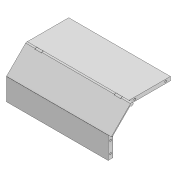
# Autodesk Inventor part: Electronics Housing Main
Saved by Autodesk Inventor 2020 (Build 240168000, 168)
## iProperties
Created: 2021-08-28
Part Number: Electronics Housing Main
Material: Generic
Document SubType Name: Modeling
Designer: Coy
Density: 1 g/cm^3
Appearance: Default
Author: Coy
Autodesk Inventor part; units mm, degrees
ref_plane "YZ Plane" through (0, 0, 0) normal (1, 0, 0) x (0, 1, 0)
ref_plane "XZ Plane" through (0, 0, 0) normal (0, 1, 0) x (-1, 0, 0)
ref_plane "XY Plane" through (0, 0, 0) normal (0, 0, 1) x (1, 0, 0)
sketch "Sketch1" plane through (0, 0, 0) normal (1, 0, 0) x (0, 1, 0)
  line L0 (1, 1) -> (56, 1) construction
  line L1 (56, 1) -> (56, 121) construction
  line L2 (56, 121) -> (1, 121) construction
  line L3 (1, 121) -> (1, 1) construction
  line L4 (80.7487, 174.033) -> (45.3934, 138.6777) construction
  line L5 (45.3934, 138.6777) -> (73.6777, 110.3934) construction
  line L6 (73.6777, 110.3934) -> (109.033, 145.7487) construction
  line L7 (109.033, 145.7487) -> (80.7487, 174.033) construction
  line L8 (59.5355, 124.5355) -> (56, 121) construction
  line L9 (0, 0) -> (125, 0) construction
  line L10 (125, 0) -> (125, 190) construction
  line L11 (125, 190) -> (0, 190) construction
  line L12 (0, 190) -> (0, 0) construction
  line L13 (109.033, 145.7487) -> (80.7487, 174.033) construction
  line L14 (80.7487, 174.033) -> (94.8909, 188.1751) construction
  line L15 (94.8909, 188.1751) -> (123.1751, 159.8909) construction
  line L16 (123.1751, 159.8909) -> (109.033, 145.7487) construction
  line L17 (125, 129.7817) -> (64.7817, 190)
  line L18 (125, 129.7817) -> (125, 0)
  line L19 (125, 0) -> (0, 0)
  line L20 (0, 0) -> (0, 190)
  line L21 (0, 190) -> (64.7817, 190)
  line L22 (66.0244, 193) -> (128, 131.0244)
  line L23 (128, 131.0244) -> (128, -3)
  line L24 (128, -3) -> (-3, -3)
  line L25 (-3, -3) -> (-3, 193)
  line L26 (-3, 193) -> (66.0244, 193)
  line L27 (128, 131.0244) -> (123.1522, 129.0164) construction
  circle A0 centre (123.1522, 129.0164) radius 2.5
  circle A1 centre (123.1522, 129.0164) radius 7.098
  point P0 (122.914, 136.1104)
  point P1 (128, 123.8317)
  dimension "d0" = 55
  dimension "d1" = 120
  dimension "d2" = 50
  dimension "d3" = 40
  dimension "d4" = 135
  dimension "d5" = 135
  dimension "d6" = 5
  dimension "d7" = 125
  dimension "d8" = 190
  dimension "d9" = 1
  dimension "d10" = 1
  dimension "d11" = 20
  dimension "d12" = 3
  dimension "d36" = 5
  dimension "d37" = 14.196
  constraints: 56 end point, 11 perpendicular, 8 parallel, 4 point on line, 2 centre point, 2 coincident, 2 horizontal, 1 collinear, 1 midpoint, 4 other
  measures "d0" distance of L2.end L1.end
  measures "d1" distance of L1.end L0.end
  measures "d2" distance of L4.start L4.end
  measures "d3" distance of L5.end L4.end
  measures "d4" angle of L1 L6
  measures "d5" angle of L1 L8
  measures "d6" distance of L8.start L1.end
  measures "d7" distance of L9.start L9.end
  measures "d8" distance of L11.end L9.start
  measures "d9" distance between parallel lines of L9 L0
  measures "d10" distance between parallel lines of L12 L3
  measures "d11" distance of L4.start L14.end
  measures "d12" distance between parallel lines of L17 L22
  measures "d36" diameter of A0
  measures "d37" diameter of A1
extrude "Extrusion1" add sketch "Sketch1" along normal blind 10
sketch "Sketch2" plane through (10, 0, 0) normal (1, 0, 0) x (0, 0, -1)
  line L0 (-193, -3) -> (3, -3) projected
  line L1 (3, -3) -> (3, 128) projected
  line L2 (3, 128) -> (-123.8317, 128) projected
  line L3 (-136.1104, 122.914) -> (-193, 66.0244) projected
  line L4 (-193, 66.0244) -> (-193, -3) projected
  line L5 (0, 125) -> (0, 0)
  line L6 (0, 0) -> (-190, 0)
  line L7 (-190, 0) -> (-190, 64.7817)
  line L8 (-193, 66.0244) -> (-193, -3) projected
  line L9 (-189.75, 64.6782) -> (-193, 66.0244)
  line L10 (-189.7704, 65.0114) -> (-192.7704, 66.254)
  line L11 (-131.0244, 128) -> (-129.0164, 123.1522) construction
  circle A0 centre (-129.0164, 123.1522) radius 2.5 construction
  circle A1 centre (-129.0164, 123.1522) radius 2.75 construction
  arc A2 (-133.4921, 121.2897) -> (-129.0164, 128) centre (-129.0164, 123.1522) ccw
  line L12 (-131.0244, 128) -> (-193, 66.0244) construction
  line L13 (-133.5692, 120.859) -> (-189.75, 64.6782)
  arc A3 (-133.5692, 120.859) -> (-127.4396, 128) centre (-129.0164, 123.1522) ccw
  line L14 (-129.7817, 125) -> (-126.9796, 125) construction
  line L15 (-124.2653, 125) -> (0, 125)
  line L16 (-190, 64.7817) -> (-133.4921, 121.2897)
  line L17 (-131.7631, 123.0186) -> (-129.7817, 125) construction
  arc A4 (-123.8317, 128) -> (-136.1104, 122.914) centre (-129.0164, 123.1522) ccw projected
  line L18 (-136.1104, 122.914) -> (-131.0244, 128)
  line L19 (3, 128) -> (-123.8317, 128) projected
  line L20 (-131.0244, 128) -> (-123.8317, 128)
  circle A5 centre (-129.0164, 123.1522) radius 4.8478
  circle A6 centre (-129.0164, 123.1522) radius 5.0978
  line L21 (0, 118.0545) -> (-129.0164, 118.0545)
  point P0 (0, 0)
  point P1 (-132.4443, 126.5801)
  dimension "d16" = 0.3
  dimension "d18" = 5
  dimension "d19" = 0.25
  constraints: 28 end point, 7 point on circle, 7 point on line, 5 centre point, 3 coincident, 2 horizontal, 2 parallel, 1 tangent, 1 vertical alignment, 5 other
  measures "d16" distance between parallel lines of L9 L10
  measures "d18" diameter of A0
  measures "d19" radial gap between concentric circles of A0 A1
extrude "Extrusion2" cut sketch "Sketch2" against normal through all contours L3 L10 L16 L9 | L16 A6 L13 L9 | L20 A6 L18 A4 | A3 A6 L16 A2 L20 | L20 A6 | A6 L18 | A5 L18 A6 L20 | A6 L18 L20
sketch "Sketch3" plane through (10, 0, 0) normal (1, 0, 0) x (0, 0, -1)
  line L0 (-193, -3) -> (3, -3)
  line L1 (3, -3) -> (3, 128)
  line L2 (3, 128) -> (-131.0244, 128)
  line L3 (-131.0244, 128) -> (-192.7704, 66.254)
  line L4 (-193, 66.0244) -> (-193, -3)
  line L5 (0, 125) -> (0, 0)
  line L6 (0, 0) -> (-190, 0)
  line L7 (-190, 0) -> (-190, 64.7817)
  line L8 (-193, 66.0244) -> (-193, -3)
  line L9 (-189.75, 64.6782) -> (-193, 66.0244)
  line L10 (-189.7704, 65.0114) -> (-192.7704, 66.254)
  line L11 (-131.0244, 128) -> (-129.0164, 123.1522) construction
  circle A0 centre (-129.0164, 123.1522) radius 2.5 construction
  circle A1 centre (-129.0164, 123.1522) radius 2.75 construction
  arc A2 (-133.4921, 121.2897) -> (-129.0164, 128) centre (-129.0164, 123.1522) ccw
  line L12 (-131.0244, 128) -> (-193, 66.0244) construction
  line L13 (-133.5692, 120.859) -> (-189.75, 64.6782)
  arc A3 (-133.5692, 120.859) -> (-127.4396, 128) centre (-129.0164, 123.1522) ccw
  line L14 (-129.7817, 125) -> (-126.9796, 125) construction
  line L15 (-122.1634, 125) -> (0, 125)
  line L16 (-189.7704, 65.0114) -> (-133.4921, 121.2897)
  line L17 (-131.7631, 123.0186) -> (-129.7817, 125) construction
  arc A4 (-135.0362, 119.392) -> (-122.1634, 125) centre (-129.0164, 123.1522) ccw
  arc A5 (-133.4921, 121.2897) -> (-132.4443, 126.5801) centre (-129.0164, 123.1522) ccw projected
  line L18 (0, 116.0545) -> (-129.0164, 116.0545)
  point P0 (0, 0)
  point P1 (0, 0)
  dimension "d25" = 0.3
  dimension "d26" = 5
  dimension "d27" = 0.25
  dimension "d28" = 2
  constraints: 38 end point, 9 point on circle, 6 point on line, 5 centre point, 2 tangent, 1 coincident, 1 horizontal, 1 parallel, 2 other
  measures "d25" distance between parallel lines of L9 L10
  measures "d26" diameter of A0
  measures "d27" radial gap between concentric circles of A0 A1
  measures "d28" radial gap between concentric circles of A3 A4
extrude "Extrusion3" add sketch "Sketch3" along normal blind 20 contours L4 L9 L7 L6 L5 L15 A4 L13 A3 L2 L1 L0 | L18 A4 L15 L5 | A2 L16 L10 L3 A5
sketch "Sketch4" plane through (30, 0, 0) normal (1, 0, 0) x (0, 0, -1)
  line L0 (-193, -3) -> (3, -3)
  line L1 (3, -3) -> (3, 128)
  line L2 (3, 128) -> (-123.8317, 128)
  line L3 (-136.1104, 122.914) -> (-193, 66.0244)
  line L4 (-193, 66.0244) -> (-193, -3)
  line L5 (0, 125) -> (0, 0)
  line L6 (0, 0) -> (-190, 0)
  line L7 (-190, 0) -> (-190, 64.7817)
  line L8 (-193, 66.0244) -> (-193, -3)
  line L9 (-189.75, 64.6782) -> (-193, 66.0244)
  line L10 (-189.7704, 65.0114) -> (-192.7704, 66.254)
  line L11 (-131.0244, 128) -> (-129.0164, 123.1522) construction
  circle A0 centre (-129.0164, 123.1522) radius 2.5
  circle A1 centre (-129.0164, 123.1522) radius 2.75 construction
  arc A2 (-133.4921, 121.2897) -> (-129.0164, 128) centre (-129.0164, 123.1522) ccw
  line L12 (-131.0244, 128) -> (-193, 66.0244) construction
  line L13 (-133.5692, 120.859) -> (-189.75, 64.6782)
  arc A3 (-133.5692, 120.859) -> (-127.4396, 128) centre (-129.0164, 123.1522) ccw
  line L14 (-129.7817, 125) -> (-126.9796, 125) construction
  line L15 (-124.2653, 125) -> (0, 125)
  line L16 (-190, 64.7817) -> (-133.4921, 121.2897)
  line L17 (-131.7631, 123.0186) -> (-129.7817, 125) construction
  arc A4 (-123.8317, 128) -> (-136.1104, 122.914) centre (-129.0164, 123.1522) ccw
  line L18 (-136.1104, 122.914) -> (-131.0244, 128)
  line L19 (3, 128) -> (-123.8317, 128)
  line L20 (-131.0244, 128) -> (-123.8317, 128)
  circle A5 centre (-129.0164, 123.1522) radius 4.8478
  circle A6 centre (-129.0164, 123.1522) radius 5.0978
  line L21 (0, 116.0545) -> (0, 0) projected
  line L22 (0, 0) -> (-190, 0) projected
  line L23 (-190, 0) -> (-190, 64.7817) projected
  line L24 (-190, 64.7817) -> (-193, 66.0244) projected
  line L25 (-193, 66.0244) -> (-193, -3) projected
  line L26 (-193, -3) -> (3, -3) projected
  line L27 (3, -3) -> (3, 128) projected
  line L28 (3, 128) -> (-127.4396, 128) projected
  arc A7 (-133.5692, 120.859) -> (-127.4396, 128) centre (-129.0164, 123.1522) ccw projected
  line L29 (-133.5692, 120.859) -> (-135.0362, 119.392) projected
  arc A8 (-135.0362, 119.392) -> (-129.0164, 116.0545) centre (-129.0164, 123.1522) ccw projected
  arc A9 (-133.4921, 121.2897) -> (-132.4443, 126.5801) centre (-129.0164, 123.1522) ccw projected
  line L30 (-132.4443, 126.5801) -> (-192.7704, 66.254) projected
  line L31 (-192.7704, 66.254) -> (-189.7704, 65.0114) projected
  line L32 (-189.7704, 65.0114) -> (-133.4921, 121.2897) projected
  line L33 (-129.0164, 116.0545) -> (0, 116.0545) projected
  point P0 (0, 0)
  point P1 (-127.4396, 128)
  point P2 (-122.1634, 125)
  point P3 (-133.6825, 121.0993)
  point P4 (-133.5592, 125.4651)
  point P5 (0, 116.0545)
  point P6 (0, 66.508)
  dimension "d38" = 0.3
  dimension "d39" = 5
  dimension "d40" = 0.25
  constraints: 42 end point, 9 point on circle, 7 centre point, 6 point on line, 3 coincident, 1 concentric, 1 horizontal, 1 parallel, 1 tangent, 2 other
  measures "d38" distance between parallel lines of L9 L10
  measures "d39" diameter of A0
  measures "d40" radial gap between concentric circles of A0 A1
extrude "Extrusion4" add sketch "Sketch4" along normal blind 0.35 contours L4 L9 L7 L6 L5 L15 A3 L20 L2 L1 L0 | L3 L18 A6 L16 L10 | L13 A3 L15 L5 L33 A8 | A0
sketch "Sketch5" plane through (30.35, 0, 0) normal (1, 0, 0) x (0, 0, -1)
  line L0 (-193, -3) -> (3, -3)
  line L1 (3, -3) -> (3, 128)
  line L2 (3, 128) -> (-123.8317, 128)
  line L3 (-136.1104, 122.914) -> (-193, 66.0244)
  line L4 (-193, 66.0244) -> (-193, -3)
  line L5 (0, 125) -> (0, 0)
  line L6 (0, 0) -> (-190, 0)
  line L7 (-190, 0) -> (-190, 64.7817)
  line L8 (-193, 66.0244) -> (-193, -3)
  line L9 (-189.75, 64.6782) -> (-193, 66.0244)
  line L10 (-189.7704, 65.0114) -> (-192.7704, 66.254)
  line L11 (-131.0244, 128) -> (-129.0164, 123.1522) construction
  circle A0 centre (-129.0164, 123.1522) radius 2.5
  circle A1 centre (-129.0164, 123.1522) radius 2.75
  arc A2 (-133.4921, 121.2897) -> (-129.0164, 128) centre (-129.0164, 123.1522) ccw
  line L12 (-131.0244, 128) -> (-193, 66.0244) construction
  line L13 (-133.5692, 120.859) -> (-189.75, 64.6782)
  arc A3 (-133.5692, 120.859) -> (-127.4396, 128) centre (-129.0164, 123.1522) ccw
  line L14 (-129.7817, 125) -> (-126.9796, 125) construction
  line L15 (-124.2653, 125) -> (0, 125)
  line L16 (-190, 64.7817) -> (-133.4921, 121.2897)
  line L17 (-131.7631, 123.0186) -> (-129.7817, 125) construction
  arc A4 (-123.8317, 128) -> (-136.1104, 122.914) centre (-129.0164, 123.1522) ccw
  line L18 (-136.1104, 122.914) -> (-131.0244, 128)
  line L19 (3, 128) -> (-123.8317, 128)
  line L20 (-131.0244, 128) -> (-123.8317, 128)
  circle A5 centre (-129.0164, 123.1522) radius 4.8478
  circle A6 centre (-129.0164, 123.1522) radius 5.0978
  line L21 (0, 125) -> (0, 0)
  line L22 (0, 0) -> (-190, 0)
  line L23 (-190, 0) -> (-190, 64.7817)
  line L24 (-190, 64.7817) -> (-193, 66.0244)
  line L25 (-193, 66.0244) -> (-193, -3)
  line L26 (-193, -3) -> (3, -3)
  line L27 (3, -3) -> (3, 128)
  line L28 (3, 128) -> (-127.4396, 128)
  arc A7 (-133.5692, 120.859) -> (-127.4396, 128) centre (-129.0164, 123.1522) ccw
  line L29 (-133.3825, 121.0457) -> (-135.0362, 119.392)
  arc A8 (-135.0362, 119.392) -> (-122.1634, 125) centre (-129.0164, 123.1522) ccw
  line L30 (-122.1634, 125) -> (0, 125)
  arc A9 (-133.4921, 121.2897) -> (-132.4443, 126.5801) centre (-129.0164, 123.1522) ccw
  line L31 (-132.4443, 126.5801) -> (-192.7704, 66.254)
  line L32 (-192.7704, 66.254) -> (-189.7704, 65.0114)
  line L33 (-189.7704, 65.0114) -> (-133.4921, 121.2897)
  line L34 (-127.4396, 128) -> (-127.5334, 127.7676)
  line L35 (-129.0164, 116.0545) -> (0, 116.0545) projected
  point P0 (0, 0)
  point P1 (0, 0)
  point P2 (-127.4396, 128)
  point P3 (-122.1634, 125)
  point P4 (-133.6825, 121.0993)
  point P5 (-133.5592, 125.4651)
  point P6 (-127.4396, 128)
  point P7 (-122.1634, 125)
  point P8 (-133.6825, 121.0993)
  point P9 (-133.5592, 125.4651)
  dimension "d43" = 0.3
  dimension "d44" = 5
  dimension "d45" = 0.25
  dimension "d46" = 112
  constraints: 70 end point, 16 point on circle, 9 centre point, 7 point on line, 3 coincident, 1 concentric, 1 horizontal, 1 parallel, 1 tangent, 5 other
  measures "d43" distance between parallel lines of L9 L10
  measures "d44" diameter of A0
  measures "d45" radial gap between concentric circles of A0 A1
  measures "d46" angle of L20 L34
extrude "Extrusion5" add sketch "Sketch5" along normal blind 20 contours L4 L9 L7 L6 L5 L15 A3 L20 L2 L1 L0 | L3 L18 A6 L16 L10 | A3 L29 A2 L34 | L13 A3 L15 A8 | A2 A5 | L35 A8 L15 L5 | A0
sketch "Sketch6" plane through (50.35, 0, 0) normal (1, 0, 0) x (0, 0, -1)
  line L0 (-193, -3) -> (3, -3)
  line L1 (3, -3) -> (3, 128)
  line L2 (3, 128) -> (-123.8317, 128)
  line L3 (-136.1104, 122.914) -> (-193, 66.0244)
  line L4 (-193, 66.0244) -> (-193, -3)
  line L5 (0, 125) -> (0, 0)
  line L6 (0, 0) -> (-190, 0)
  line L7 (-190, 0) -> (-190, 64.7817)
  line L8 (-193, 66.0244) -> (-193, -3)
  line L9 (-189.75, 64.6782) -> (-193, 66.0244)
  line L10 (-189.7704, 65.0114) -> (-192.7704, 66.254)
  line L11 (-131.0244, 128) -> (-129.0164, 123.1522) construction
  circle A0 centre (-129.0164, 123.1522) radius 2.5
  circle A1 centre (-129.0164, 123.1522) radius 2.75
  arc A2 (-133.4921, 121.2897) -> (-129.0164, 128) centre (-129.0164, 123.1522) ccw
  line L12 (-131.0244, 128) -> (-193, 66.0244) construction
  line L13 (-133.5692, 120.859) -> (-189.75, 64.6782)
  arc A3 (-133.5692, 120.859) -> (-127.4396, 128) centre (-129.0164, 123.1522) ccw
  line L14 (-129.7817, 125) -> (-126.9796, 125) construction
  line L15 (-124.2653, 125) -> (0, 125)
  line L16 (-190, 64.7817) -> (-133.4921, 121.2897)
  line L17 (-131.7631, 123.0186) -> (-129.7817, 125) construction
  arc A4 (-123.8317, 128) -> (-136.1104, 122.914) centre (-129.0164, 123.1522) ccw
  line L18 (-136.1104, 122.914) -> (-131.0244, 128)
  line L19 (3, 128) -> (-123.8317, 128)
  line L20 (-131.0244, 128) -> (-123.8317, 128)
  circle A5 centre (-129.0164, 123.1522) radius 4.8478
  circle A6 centre (-129.0164, 123.1522) radius 5.0978
  line L21 (0, 125) -> (0, 0)
  line L22 (0, 0) -> (-190, 0)
  line L23 (-190, 0) -> (-190, 64.7817)
  line L24 (-190, 64.7817) -> (-193, 66.0244)
  line L25 (-193, 66.0244) -> (-193, -3)
  line L26 (-193, -3) -> (3, -3)
  line L27 (3, -3) -> (3, 128)
  line L28 (3, 128) -> (-127.4396, 128)
  arc A7 (-133.5692, 120.859) -> (-127.4396, 128) centre (-129.0164, 123.1522) ccw
  line L29 (-133.3825, 121.0457) -> (-135.0362, 119.392)
  arc A8 (-135.0362, 119.392) -> (-122.1634, 125) centre (-129.0164, 123.1522) ccw
  line L30 (-122.1634, 125) -> (0, 125)
  arc A9 (-133.4921, 121.2897) -> (-132.4443, 126.5801) centre (-129.0164, 123.1522) ccw
  line L31 (-132.4443, 126.5801) -> (-192.7704, 66.254)
  line L32 (-192.7704, 66.254) -> (-189.7704, 65.0114)
  line L33 (-189.7704, 65.0114) -> (-133.4921, 121.2897)
  line L34 (-127.4396, 128) -> (-127.5334, 127.7676)
  line L35 (-129.0164, 116.0545) -> (0, 116.0545) projected
  point P0 (0, 0)
  point P1 (0, 0)
  point P2 (0, 0)
  point P3 (-127.4396, 128)
  point P4 (-122.1634, 125)
  point P5 (-133.6825, 121.0993)
  point P6 (-133.5592, 125.4651)
  point P7 (-127.4396, 128)
  point P8 (-122.1634, 125)
  point P9 (-133.6825, 121.0993)
  point P10 (-133.5592, 125.4651)
  point P11 (-127.4396, 128)
  point P12 (-122.1634, 125)
  point P13 (-133.6825, 121.0993)
  point P14 (-133.5592, 125.4651)
  dimension "d49" = 0.3
  dimension "d50" = 5
  dimension "d51" = 0.25
  dimension "d52" = 112
  constraints: 70 end point, 16 point on circle, 9 centre point, 7 point on line, 3 coincident, 1 concentric, 1 horizontal, 1 parallel, 1 tangent, 5 other
  measures "d49" distance between parallel lines of L9 L10
  measures "d50" diameter of A0
  measures "d51" radial gap between concentric circles of A0 A1
  measures "d52" angle of L20 L34
extrude "Extrusion6" add sketch "Sketch6" along normal blind 0.35 contours L4 L9 L7 L6 L5 L15 A3 L20 L2 L1 L0 | L3 L18 A6 L16 L10 | L13 A3 L15 A8 | L35 A8 L15 L5 | A0
sketch "Sketch7" plane through (50.7, 0, 0) normal (1, 0, 0) x (0, 0, -1)
  line L0 (-193, -3) -> (3, -3)
  line L1 (3, -3) -> (3, 128)
  line L2 (3, 128) -> (-123.8317, 128)
  line L3 (-136.1104, 122.914) -> (-193, 66.0244)
  line L4 (-193, 66.0244) -> (-193, -3)
  line L5 (0, 125) -> (0, 0)
  line L6 (0, 0) -> (-190, 0)
  line L7 (-190, 0) -> (-190, 64.7817)
  line L8 (-193, 66.0244) -> (-193, -3)
  line L9 (-189.75, 64.6782) -> (-193, 66.0244)
  line L10 (-189.7704, 65.0114) -> (-192.7704, 66.254)
  line L11 (-131.0244, 128) -> (-129.0164, 123.1522) construction
  circle A0 centre (-129.0164, 123.1522) radius 2.5
  circle A1 centre (-129.0164, 123.1522) radius 2.75
  arc A2 (-133.4921, 121.2897) -> (-129.0164, 128) centre (-129.0164, 123.1522) ccw
  line L12 (-131.0244, 128) -> (-193, 66.0244) construction
  line L13 (-133.5692, 120.859) -> (-189.75, 64.6782)
  arc A3 (-133.5692, 120.859) -> (-127.4396, 128) centre (-129.0164, 123.1522) ccw
  line L14 (-129.7817, 125) -> (-126.9796, 125) construction
  line L15 (-124.2653, 125) -> (0, 125)
  line L16 (-190, 64.7817) -> (-133.4921, 121.2897)
  line L17 (-131.7631, 123.0186) -> (-129.7817, 125) construction
  arc A4 (-123.8317, 128) -> (-136.1104, 122.914) centre (-129.0164, 123.1522) ccw
  line L18 (-136.1104, 122.914) -> (-131.0244, 128)
  line L19 (3, 128) -> (-123.8317, 128)
  line L20 (-131.0244, 128) -> (-123.8317, 128)
  circle A5 centre (-129.0164, 123.1522) radius 4.8478
  circle A6 centre (-129.0164, 123.1522) radius 5.0978
  line L21 (0, 125) -> (0, 0)
  line L22 (0, 0) -> (-190, 0)
  line L23 (-190, 0) -> (-190, 64.7817)
  line L24 (-190, 64.7817) -> (-193, 66.0244)
  line L25 (-193, 66.0244) -> (-193, -3)
  line L26 (-193, -3) -> (3, -3)
  line L27 (3, -3) -> (3, 128)
  line L28 (3, 128) -> (-127.4396, 128)
  arc A7 (-133.5692, 120.859) -> (-127.4396, 128) centre (-129.0164, 123.1522) ccw
  line L29 (-133.3825, 121.0457) -> (-135.0362, 119.392)
  arc A8 (-135.0362, 119.392) -> (-122.1634, 125) centre (-129.0164, 123.1522) ccw
  line L30 (-122.1634, 125) -> (0, 125)
  arc A9 (-133.4921, 121.2897) -> (-132.4443, 126.5801) centre (-129.0164, 123.1522) ccw
  line L31 (-132.4443, 126.5801) -> (-192.7704, 66.254)
  line L32 (-192.7704, 66.254) -> (-189.7704, 65.0114)
  line L33 (-189.7704, 65.0114) -> (-133.4921, 121.2897)
  line L34 (-127.4396, 128) -> (-127.5334, 127.7676)
  line L35 (-129.0164, 116.0545) -> (0, 116.0545) projected
  point P0 (0, 0)
  point P1 (0, 0)
  point P2 (0, 0)
  point P3 (0, 0)
  point P4 (-127.4396, 128)
  point P5 (-122.1634, 125)
  point P6 (-133.6825, 121.0993)
  point P7 (-133.5592, 125.4651)
  point P8 (-127.4396, 128)
  point P9 (-122.1634, 125)
  point P10 (-133.6825, 121.0993)
  point P11 (-133.5592, 125.4651)
  point P12 (-127.4396, 128)
  point P13 (-122.1634, 125)
  point P14 (-133.6825, 121.0993)
  point P15 (-133.5592, 125.4651)
  point P16 (-127.4396, 128)
  point P17 (-122.1634, 125)
  dimension "d55" = 0.3
  dimension "d56" = 5
  dimension "d57" = 0.25
  dimension "d58" = 112
  constraints: 70 end point, 16 point on circle, 9 centre point, 7 point on line, 3 coincident, 1 concentric, 1 horizontal, 1 parallel, 1 tangent, 5 other
  measures "d55" distance between parallel lines of L9 L10
  measures "d56" diameter of A0
  measures "d57" radial gap between concentric circles of A0 A1
  measures "d58" angle of L20 L34
extrude "Extrusion7" add sketch "Sketch7" along normal blind 228.6 contours L4 L9 L7 L6 L5 L15 A3 L20 L2 L1 L0 | L3 L18 A6 L16 L10 | L18 A5 L16 A6 | L13 A3 L15 A8 | A2 A5 | L35 A8 L15 L5 | A0 | A1
sketch "Sketch8" plane through (279.3, 0, 0) normal (1, 0, 0) x (0, 0, -1)
  line L0 (-193, -3) -> (3, -3)
  line L1 (3, -3) -> (3, 128)
  line L2 (3, 128) -> (-123.8317, 128)
  line L3 (-136.1104, 122.914) -> (-193, 66.0244)
  line L4 (-193, 66.0244) -> (-193, -3)
  line L5 (0, 125) -> (0, 0)
  line L6 (0, 0) -> (-190, 0)
  line L7 (-190, 0) -> (-190, 64.7817)
  line L8 (-193, 66.0244) -> (-193, -3)
  line L9 (-189.75, 64.6782) -> (-193, 66.0244)
  line L10 (-189.7704, 65.0114) -> (-192.7704, 66.254)
  line L11 (-131.0244, 128) -> (-129.0164, 123.1522) construction
  circle A0 centre (-129.0164, 123.1522) radius 2.5
  circle A1 centre (-129.0164, 123.1522) radius 2.75
  arc A2 (-133.4921, 121.2897) -> (-129.0164, 128) centre (-129.0164, 123.1522) ccw
  line L12 (-131.0244, 128) -> (-193, 66.0244) construction
  line L13 (-133.5692, 120.859) -> (-189.75, 64.6782)
  arc A3 (-133.5692, 120.859) -> (-127.4396, 128) centre (-129.0164, 123.1522) ccw
  line L14 (-129.7817, 125) -> (-126.9796, 125) construction
  line L15 (-124.2653, 125) -> (0, 125)
  line L16 (-190, 64.7817) -> (-133.4921, 121.2897)
  line L17 (-131.7631, 123.0186) -> (-129.7817, 125) construction
  arc A4 (-123.8317, 128) -> (-136.1104, 122.914) centre (-129.0164, 123.1522) ccw
  line L18 (-136.1104, 122.914) -> (-131.0244, 128)
  line L19 (3, 128) -> (-123.8317, 128)
  line L20 (-131.0244, 128) -> (-123.8317, 128)
  circle A5 centre (-129.0164, 123.1522) radius 4.8478
  circle A6 centre (-129.0164, 123.1522) radius 5.0978
  line L21 (0, 125) -> (0, 0)
  line L22 (0, 0) -> (-190, 0)
  line L23 (-190, 0) -> (-190, 64.7817)
  line L24 (-190, 64.7817) -> (-193, 66.0244)
  line L25 (-193, 66.0244) -> (-193, -3)
  line L26 (-193, -3) -> (3, -3)
  line L27 (3, -3) -> (3, 128)
  line L28 (3, 128) -> (-127.4396, 128)
  arc A7 (-133.5692, 120.859) -> (-127.4396, 128) centre (-129.0164, 123.1522) ccw
  line L29 (-133.3825, 121.0457) -> (-135.0362, 119.392)
  arc A8 (-135.0362, 119.392) -> (-122.1634, 125) centre (-129.0164, 123.1522) ccw
  line L30 (-122.1634, 125) -> (0, 125)
  arc A9 (-133.4921, 121.2897) -> (-132.4443, 126.5801) centre (-129.0164, 123.1522) ccw
  line L31 (-132.4443, 126.5801) -> (-192.7704, 66.254)
  line L32 (-192.7704, 66.254) -> (-189.7704, 65.0114)
  line L33 (-189.7704, 65.0114) -> (-133.4921, 121.2897)
  line L34 (-127.4396, 128) -> (-127.5334, 127.7676)
  line L35 (-129.0164, 116.0545) -> (0, 116.0545) projected
  point P0 (0, 0)
  point P1 (0, 0)
  point P2 (0, 0)
  point P3 (0, 0)
  point P4 (-127.4396, 128)
  point P5 (-122.1634, 125)
  point P6 (-133.6825, 121.0993)
  point P7 (-133.5592, 125.4651)
  point P8 (-127.4396, 128)
  point P9 (-122.1634, 125)
  point P10 (-133.6825, 121.0993)
  point P11 (-133.5592, 125.4651)
  point P12 (-127.4396, 128)
  point P13 (-122.1634, 125)
  point P14 (-133.6825, 121.0993)
  point P15 (-133.5592, 125.4651)
  point P16 (-133.6825, 121.0993)
  point P17 (-133.5592, 125.4651)
  point P18 (-127.4396, 128)
  point P19 (-122.1634, 125)
  dimension "d61" = 0.3
  dimension "d62" = 5
  dimension "d63" = 0.25
  dimension "d64" = 112
  constraints: 70 end point, 16 point on circle, 9 centre point, 7 point on line, 3 coincident, 1 concentric, 1 horizontal, 1 parallel, 1 tangent, 5 other
  measures "d61" distance between parallel lines of L9 L10
  measures "d62" diameter of A0
  measures "d63" radial gap between concentric circles of A0 A1
  measures "d64" angle of L20 L34
extrude "Extrusion8" add sketch "Sketch8" along normal blind 0.35 contours L4 L9 L7 L6 L5 L15 A3 L20 L2 L1 L0 | L3 L18 A6 L16 L10 | L13 A3 L15 A8 | L35 A8 L15 L5 | A0
sketch "Sketch9" plane through (279.65, 0, 0) normal (1, 0, 0) x (0, 0, -1)
  line L0 (-193, -3) -> (3, -3)
  line L1 (3, -3) -> (3, 128)
  line L2 (3, 128) -> (-123.8317, 128)
  line L3 (-136.1104, 122.914) -> (-193, 66.0244)
  line L4 (-193, 66.0244) -> (-193, -3)
  line L5 (0, 125) -> (0, 0)
  line L6 (0, 0) -> (-190, 0)
  line L7 (-190, 0) -> (-190, 64.7817)
  line L8 (-193, 66.0244) -> (-193, -3)
  line L9 (-189.75, 64.6782) -> (-193, 66.0244)
  line L10 (-189.7704, 65.0114) -> (-192.7704, 66.254)
  line L11 (-131.0244, 128) -> (-129.0164, 123.1522) construction
  circle A0 centre (-129.0164, 123.1522) radius 2.5
  circle A1 centre (-129.0164, 123.1522) radius 2.75
  arc A2 (-133.4921, 121.2897) -> (-129.0164, 128) centre (-129.0164, 123.1522) ccw
  line L12 (-131.0244, 128) -> (-193, 66.0244) construction
  line L13 (-133.5692, 120.859) -> (-189.75, 64.6782)
  arc A3 (-133.5692, 120.859) -> (-127.4396, 128) centre (-129.0164, 123.1522) ccw
  line L14 (-129.7817, 125) -> (-126.9796, 125) construction
  line L15 (-124.2653, 125) -> (0, 125)
  line L16 (-190, 64.7817) -> (-133.4921, 121.2897)
  line L17 (-131.7631, 123.0186) -> (-129.7817, 125) construction
  arc A4 (-123.8317, 128) -> (-136.1104, 122.914) centre (-129.0164, 123.1522) ccw
  line L18 (-136.1104, 122.914) -> (-131.0244, 128)
  line L19 (3, 128) -> (-123.8317, 128)
  line L20 (-131.0244, 128) -> (-123.8317, 128)
  circle A5 centre (-129.0164, 123.1522) radius 4.8478
  circle A6 centre (-129.0164, 123.1522) radius 5.0978
  line L21 (0, 125) -> (0, 0)
  line L22 (0, 0) -> (-190, 0)
  line L23 (-190, 0) -> (-190, 64.7817)
  line L24 (-190, 64.7817) -> (-193, 66.0244)
  line L25 (-193, 66.0244) -> (-193, -3)
  line L26 (-193, -3) -> (3, -3)
  line L27 (3, -3) -> (3, 128)
  line L28 (3, 128) -> (-127.4396, 128)
  arc A7 (-133.5692, 120.859) -> (-127.4396, 128) centre (-129.0164, 123.1522) ccw
  line L29 (-133.3825, 121.0457) -> (-135.0362, 119.392)
  arc A8 (-135.0362, 119.392) -> (-122.1634, 125) centre (-129.0164, 123.1522) ccw
  line L30 (-122.1634, 125) -> (0, 125)
  arc A9 (-133.4921, 121.2897) -> (-132.4443, 126.5801) centre (-129.0164, 123.1522) ccw
  line L31 (-132.4443, 126.5801) -> (-192.7704, 66.254)
  line L32 (-192.7704, 66.254) -> (-189.7704, 65.0114)
  line L33 (-189.7704, 65.0114) -> (-133.4921, 121.2897)
  line L34 (-127.4396, 128) -> (-127.5334, 127.7676)
  line L35 (-129.0164, 116.0545) -> (0, 116.0545) projected
  point P0 (0, 0)
  point P1 (0, 0)
  point P2 (0, 0)
  point P3 (0, 0)
  point P4 (0, 0)
  point P5 (-127.4396, 128)
  point P6 (-122.1634, 125)
  point P7 (-133.6825, 121.0993)
  point P8 (-133.5592, 125.4651)
  point P9 (-127.4396, 128)
  point P10 (-122.1634, 125)
  point P11 (-133.6825, 121.0993)
  point P12 (-133.5592, 125.4651)
  point P13 (-127.4396, 128)
  point P14 (-122.1634, 125)
  point P15 (-133.6825, 121.0993)
  point P16 (-133.5592, 125.4651)
  point P17 (-133.6825, 121.0993)
  point P18 (-133.5592, 125.4651)
  point P19 (-127.4396, 128)
  point P20 (-122.1634, 125)
  point P21 (-133.6825, 121.0993)
  point P22 (-133.5592, 125.4651)
  point P23 (-127.4396, 128)
  point P24 (-122.1634, 125)
  dimension "d67" = 0.3
  dimension "d68" = 5
  dimension "d69" = 0.25
  dimension "d70" = 112
  constraints: 70 end point, 16 point on circle, 9 centre point, 7 point on line, 3 coincident, 1 concentric, 1 horizontal, 1 parallel, 1 tangent, 5 other
  measures "d67" distance between parallel lines of L9 L10
  measures "d68" diameter of A0
  measures "d69" radial gap between concentric circles of A0 A1
  measures "d70" angle of L20 L34
extrude "Extrusion9" add sketch "Sketch9" along normal blind 20 contours L4 L9 L7 L6 L5 L15 A3 L20 L2 L1 L0 | L3 L18 A6 L16 L10 | A3 L29 A2 L34 | L13 A3 L15 A8 | A2 A5 | L35 A8 L15 L5 | A0
sketch "Sketch10" plane through (299.65, 0, 0) normal (1, 0, 0) x (0, 0, -1)
  line L0 (-193, -3) -> (3, -3)
  line L1 (3, -3) -> (3, 128)
  line L2 (3, 128) -> (-123.8317, 128)
  line L3 (-136.1104, 122.914) -> (-193, 66.0244)
  line L4 (-193, 66.0244) -> (-193, -3)
  line L5 (0, 125) -> (0, 0)
  line L6 (0, 0) -> (-190, 0)
  line L7 (-190, 0) -> (-190, 64.7817)
  line L8 (-193, 66.0244) -> (-193, -3)
  line L9 (-189.75, 64.6782) -> (-193, 66.0244)
  line L10 (-189.7704, 65.0114) -> (-192.7704, 66.254)
  line L11 (-131.0244, 128) -> (-129.0164, 123.1522) construction
  circle A0 centre (-129.0164, 123.1522) radius 2.5
  circle A1 centre (-129.0164, 123.1522) radius 2.75
  arc A2 (-133.4921, 121.2897) -> (-129.0164, 128) centre (-129.0164, 123.1522) ccw
  line L12 (-131.0244, 128) -> (-193, 66.0244) construction
  line L13 (-133.5692, 120.859) -> (-189.75, 64.6782)
  arc A3 (-133.5692, 120.859) -> (-127.4396, 128) centre (-129.0164, 123.1522) ccw
  line L14 (-129.7817, 125) -> (-126.9796, 125) construction
  line L15 (-124.2653, 125) -> (0, 125)
  line L16 (-190, 64.7817) -> (-133.4921, 121.2897)
  line L17 (-131.7631, 123.0186) -> (-129.7817, 125) construction
  arc A4 (-123.8317, 128) -> (-136.1104, 122.914) centre (-129.0164, 123.1522) ccw
  line L18 (-136.1104, 122.914) -> (-131.0244, 128)
  line L19 (3, 128) -> (-123.8317, 128)
  line L20 (-131.0244, 128) -> (-123.8317, 128)
  circle A5 centre (-129.0164, 123.1522) radius 4.8478
  circle A6 centre (-129.0164, 123.1522) radius 5.0978
  line L21 (0, 125) -> (0, 0)
  line L22 (0, 0) -> (-190, 0)
  line L23 (-190, 0) -> (-190, 64.7817)
  line L24 (-190, 64.7817) -> (-193, 66.0244)
  line L25 (-193, 66.0244) -> (-193, -3)
  line L26 (-193, -3) -> (3, -3)
  line L27 (3, -3) -> (3, 128)
  line L28 (3, 128) -> (-127.4396, 128)
  arc A7 (-133.5692, 120.859) -> (-127.4396, 128) centre (-129.0164, 123.1522) ccw
  line L29 (-133.3825, 121.0457) -> (-135.0362, 119.392)
  arc A8 (-135.0362, 119.392) -> (-122.1634, 125) centre (-129.0164, 123.1522) ccw
  line L30 (-122.1634, 125) -> (0, 125)
  arc A9 (-133.4921, 121.2897) -> (-132.4443, 126.5801) centre (-129.0164, 123.1522) ccw
  line L31 (-132.4443, 126.5801) -> (-192.7704, 66.254)
  line L32 (-192.7704, 66.254) -> (-189.7704, 65.0114)
  line L33 (-189.7704, 65.0114) -> (-133.4921, 121.2897)
  line L34 (-127.4396, 128) -> (-127.5334, 127.7676)
  line L35 (-129.0164, 116.0545) -> (0, 116.0545) projected
  point P0 (0, 0)
  point P1 (0, 0)
  point P2 (0, 0)
  point P3 (0, 0)
  point P4 (0, 0)
  point P5 (-127.4396, 128)
  point P6 (-122.1634, 125)
  point P7 (-133.6825, 121.0993)
  point P8 (-133.5592, 125.4651)
  point P9 (-127.4396, 128)
  point P10 (-122.1634, 125)
  point P11 (-133.6825, 121.0993)
  point P12 (-133.5592, 125.4651)
  point P13 (-127.4396, 128)
  point P14 (-122.1634, 125)
  point P15 (-133.6825, 121.0993)
  point P16 (-133.5592, 125.4651)
  point P17 (-133.6825, 121.0993)
  point P18 (-133.5592, 125.4651)
  point P19 (-127.4396, 128)
  point P20 (-122.1634, 125)
  point P21 (-133.6825, 121.0993)
  point P22 (-133.5592, 125.4651)
  point P23 (-127.4396, 128)
  point P24 (-122.1634, 125)
  dimension "d73" = 0.3
  dimension "d74" = 5
  dimension "d75" = 0.25
  dimension "d76" = 112
  constraints: 70 end point, 16 point on circle, 9 centre point, 7 point on line, 3 coincident, 1 concentric, 1 horizontal, 1 parallel, 1 tangent, 5 other
  measures "d73" distance between parallel lines of L9 L10
  measures "d74" diameter of A0
  measures "d75" radial gap between concentric circles of A0 A1
  measures "d76" angle of L20 L34
extrude "Extrusion10" add sketch "Sketch10" along normal blind 0.35 contours L4 L9 L7 L6 L5 L15 A3 L20 L2 L1 L0 | L3 L18 A6 L16 L10 | L13 A3 L15 A8 | L35 A8 L15 L5 | A0
sketch "Sketch11" plane through (300, 0, 0) normal (1, 0, 0) x (0, 0, -1)
  line L0 (-193, -3) -> (3, -3)
  line L1 (3, -3) -> (3, 128)
  line L2 (3, 128) -> (-123.8317, 128)
  line L3 (-136.1104, 122.914) -> (-193, 66.0244)
  line L4 (-193, 66.0244) -> (-193, -3)
  line L5 (0, 125) -> (0, 0)
  line L6 (0, 0) -> (-190, 0)
  line L7 (-190, 0) -> (-190, 64.7817)
  line L8 (-193, 66.0244) -> (-193, -3)
  line L9 (-189.75, 64.6782) -> (-193, 66.0244)
  line L10 (-189.7704, 65.0114) -> (-192.7704, 66.254)
  line L11 (-131.0244, 128) -> (-129.0164, 123.1522) construction
  circle A0 centre (-129.0164, 123.1522) radius 2.5
  circle A1 centre (-129.0164, 123.1522) radius 2.75
  arc A2 (-133.4921, 121.2897) -> (-129.0164, 128) centre (-129.0164, 123.1522) ccw
  line L12 (-131.0244, 128) -> (-193, 66.0244) construction
  line L13 (-133.5692, 120.859) -> (-189.75, 64.6782)
  arc A3 (-133.5692, 120.859) -> (-127.4396, 128) centre (-129.0164, 123.1522) ccw
  line L14 (-129.7817, 125) -> (-126.9796, 125) construction
  line L15 (-124.2653, 125) -> (0, 125)
  line L16 (-190, 64.7817) -> (-133.4921, 121.2897)
  line L17 (-131.7631, 123.0186) -> (-129.7817, 125) construction
  arc A4 (-123.8317, 128) -> (-136.1104, 122.914) centre (-129.0164, 123.1522) ccw
  line L18 (-136.1104, 122.914) -> (-131.0244, 128)
  line L19 (3, 128) -> (-123.8317, 128)
  line L20 (-131.0244, 128) -> (-123.8317, 128)
  circle A5 centre (-129.0164, 123.1522) radius 4.8478
  circle A6 centre (-129.0164, 123.1522) radius 5.0978
  line L21 (0, 125) -> (0, 0)
  line L22 (0, 0) -> (-190, 0)
  line L23 (-190, 0) -> (-190, 64.7817)
  line L24 (-190, 64.7817) -> (-193, 66.0244)
  line L25 (-193, 66.0244) -> (-193, -3)
  line L26 (-193, -3) -> (3, -3)
  line L27 (3, -3) -> (3, 128)
  line L28 (3, 128) -> (-127.4396, 128)
  arc A7 (-133.5692, 120.859) -> (-127.4396, 128) centre (-129.0164, 123.1522) ccw
  line L29 (-133.3825, 121.0457) -> (-135.0362, 119.392)
  arc A8 (-135.0362, 119.392) -> (-122.1634, 125) centre (-129.0164, 123.1522) ccw
  line L30 (-122.1634, 125) -> (0, 125)
  arc A9 (-133.4921, 121.2897) -> (-132.4443, 126.5801) centre (-129.0164, 123.1522) ccw
  line L31 (-132.4443, 126.5801) -> (-192.7704, 66.254)
  line L32 (-192.7704, 66.254) -> (-189.7704, 65.0114)
  line L33 (-189.7704, 65.0114) -> (-133.4921, 121.2897)
  line L34 (-127.4396, 128) -> (-127.5334, 127.7676)
  line L35 (-129.0164, 116.0545) -> (0, 116.0545) projected
  point P0 (0, 0)
  point P1 (0, 0)
  point P2 (0, 0)
  point P3 (0, 0)
  point P4 (0, 0)
  point P5 (-127.4396, 128)
  point P6 (-122.1634, 125)
  point P7 (-133.6825, 121.0993)
  point P8 (-133.5592, 125.4651)
  point P9 (-127.4396, 128)
  point P10 (-122.1634, 125)
  point P11 (-133.6825, 121.0993)
  point P12 (-133.5592, 125.4651)
  point P13 (-127.4396, 128)
  point P14 (-122.1634, 125)
  point P15 (-133.6825, 121.0993)
  point P16 (-133.5592, 125.4651)
  point P17 (-133.6825, 121.0993)
  point P18 (-133.5592, 125.4651)
  point P19 (-127.4396, 128)
  point P20 (-122.1634, 125)
  point P21 (-127.4396, 128)
  point P22 (-122.1634, 125)
  dimension "d79" = 0.3
  dimension "d80" = 5
  dimension "d81" = 0.25
  dimension "d82" = 112
  constraints: 70 end point, 16 point on circle, 9 centre point, 7 point on line, 3 coincident, 1 concentric, 1 horizontal, 1 parallel, 1 tangent, 5 other
  measures "d79" distance between parallel lines of L9 L10
  measures "d80" diameter of A0
  measures "d81" radial gap between concentric circles of A0 A1
  measures "d82" angle of L20 L34
extrude "Extrusion11" add sketch "Sketch11" along normal blind 20 contours L4 L9 L7 L6 L5 L15 A3 L20 L2 L1 L0 | L3 L18 A6 L16 L10 | L18 A5 L16 A6 | L13 A3 L15 A8 | A2 A5 | L35 A8 L15 L5 | A0 | A1
sketch "Sketch17" plane through (320, 0, 0) normal (1, 0, 0) x (0, 0, -1)
  line L0 (-132.4443, 126.5801) -> (-192.7704, 66.254) projected
  line L1 (-192.7704, 66.254) -> (-189.7704, 65.0114) projected
  line L2 (-189.7704, 65.0114) -> (-133.4921, 121.2897) projected
  arc A0 (-133.4921, 121.2897) -> (-132.4443, 126.5801) centre (-129.0164, 123.1522) ccw projected
  point P0 (0, 0)
extrude "Extrusion17" add sketch "Sketch17" along normal blind 10
sketch "Sketch18" plane through (320, 0, 0) normal (1, 0, 0) x (0, 0, -1)
  line L0 (-190, 0) -> (-190, 64.7817) projected
  line L1 (-178, 0) -> (-178, 59.8112)
  line L2 (-135.0362, 119.392) -> (-189.75, 64.6782) projected
  line L3 (-189.75, 64.6782) -> (-178, 59.8112)
  line L4 (-190, 64.7817) -> (-193, 66.0244) projected
  line L5 (0, 0) -> (-190, 0) projected
  line L6 (-190, 64.7817) -> (-193, 66.0244) projected
  line L7 (-189.75, 64.6782) -> (-190, 64.7817)
  dimension "d109" = 12
  constraints: 6 end point, 2 collinear, 1 parallel
  measures "d109" distance between parallel lines of L0 L1
extrude "Extrusion18" add sketch "Sketch18" against normal up to surface (310 mm away)
sketch "Sketch19" plane through (320, 0, 0) normal (1, 0, 0) x (0, 0, -1)
  line L0 (-193, -3) -> (3, -3) projected
  line L1 (3, -3) -> (3, 128) projected
  line L2 (3, 128) -> (-127.4396, 128) projected
  arc A0 (-133.5692, 120.859) -> (-127.4396, 128) centre (-129.0164, 123.1522) ccw projected
  line L3 (-133.5692, 120.859) -> (-135.0362, 119.392) projected
  arc A1 (-135.0362, 119.392) -> (-129.0164, 116.0545) centre (-129.0164, 123.1522) ccw projected
  line L4 (-129.0164, 116.0545) -> (0, 116.0545) projected
  line L5 (0, 116.0545) -> (0, 0) projected
  line L6 (0, 0) -> (-178, 0) projected
  line L7 (-178, 0) -> (-178, 59.8112) projected
  line L8 (-178, 59.8112) -> (-193, 66.0244) projected
  line L9 (-193, 66.0244) -> (-193, -3) projected
  line L10 (0, 116.0545) -> (-129.0164, 116.0545) projected
  line L11 (0, 116.0545) -> (3, 116.0545)
  line L12 (3, -3) -> (3, 128) projected
  line L13 (-178, 0) -> (0, 0) projected
  line L14 (-178, 0) -> (-178, -3)
  line L15 (-193, -3) -> (3, -3) projected
  constraints: 4 end point, 2 point on line, 1 horizontal, 1 perpendicular
extrude "Extrusion19" cut sketch "Sketch19" against normal up to surface (310 mm away) contours L14 L6 L5 L11 L1 L0
sketch "Sketch20" plane through (0, -3, -3) normal (0, 0, -1) x (-1, 0, 0)
  line L0 (94.5749, 12) -> (-370.7982, 12) construction
  line L1 (0, 0) -> (-10, 0) construction
  line L2 (-10, 0) -> (-10, 62.8112) projected
  line L3 (-10, 8.75) -> (-5, 8.75)
  line L4 (-5, 8.75) -> (-5, 3.25)
  line L5 (-5, 3.25) -> (-10, 3.25)
  line L6 (-10, 3.25) -> (-10, 8.75)
  point P0 (0, 3)
  dimension "d114" = 12
  dimension "d115" = 5.5
  dimension "d116" = 3.25
  constraints: 10 end point, 2 horizontal, 2 parallel, 1 perpendicular, 1 point on line
  measures "d114" distance between parallel lines of L1 L0
  measures "d115" distance of L3.end L4.end
  measures "d116" distance between parallel lines of L0 L3
extrude "Extrusion20" cut sketch "Sketch20" against normal up to surface (181 mm away)
sketch "Sketch21" plane through (320, 0, 0) normal (1, 0, 0) x (0, 0, -1)
  line L0 (-129.0164, 116.0545) -> (3, 116.0545) construction
  line L1 (3, 116.0545) -> (3, 128) construction
  line L2 (3, 128) -> (-127.4396, 128) construction
  arc A0 (-133.5692, 120.859) -> (-127.4396, 128) centre (-129.0164, 123.1522) ccw construction
  line L3 (-133.5692, 120.859) -> (-135.0362, 119.392) construction
  arc A1 (-135.0362, 119.392) -> (-129.0164, 116.0545) centre (-129.0164, 123.1522) ccw construction
  line L4 (-178, -3) -> (-178, 59.8112) construction
  line L5 (-178, 59.8112) -> (-193, 66.0244) construction
  line L6 (-193, 66.0244) -> (-193, -3) construction
  line L7 (-193, -3) -> (-178, -3) construction
  line L8 (3, 122.0272) -> (-124.0443, 122.0272)
  arc A2 (-133.5692, 120.859) -> (-127.4396, 128) centre (-129.0164, 123.1522) ccw projected
  line L9 (-193, -3) -> (3, -3) projected
  line L10 (-185.5, -3) -> (-185.5, 62.9178)
  line L11 (-189.75, 64.6782) -> (-178, 59.8112) projected
  circle A3 centre (-12, 122.0272) radius 3
  circle A4 centre (-109.0443, 122.0272) radius 3
  circle A5 centre (-185.5, 12) radius 3
  circle A6 centre (-185.5, 47.9178) radius 3
  point P0 (0, 0)
  dimension "d119" = 6
  dimension "d120" = 15
  dimension "d121" = 6
  dimension "d122" = 15
  dimension "d123" = 6
  dimension "d124" = 6
  dimension "d125" = 15
  dimension "d126" = 15
  constraints: 6 point on line, 4 centre point, 4 end point, 1 horizontal, 1 midpoint, 1 perpendicular, 1 point on circle
  measures "d119" diameter of A3
  measures "d120" distance of L8.start A3.centre
  measures "d121" diameter of A4
  measures "d122" distance of L8.end A4.centre
  measures "d123" diameter of A6
  measures "d124" diameter of A5
  measures "d125" distance from line of L7 A5.centre
  measures "d126" distance of L10.end A6.centre
extrude "Extrusion21" cut sketch "Sketch21" against normal blind 4
sketch "Sketch22" plane through (316, 122.0272, 109.0443) normal (1, 0, 0) x (0, 0, -1)
  circle A0 centre (0, 0) radius 3 projected
  circle A1 centre (97.0443, 0) radius 3 projected
  circle A2 centre (-76.4557, -74.1095) radius 3 projected
  circle A3 centre (-76.4557, -110.0272) radius 3 projected
  circle A4 centre (-76.4557, -110.0272) radius 3 projected
  circle A5 centre (-76.4557, -110.0272) radius 2.1
  circle A6 centre (-76.4557, -74.1095) radius 3 projected
  circle A7 centre (-76.4557, -74.1095) radius 2.1
  circle A8 centre (0, 0) radius 3 projected
  circle A9 centre (0, 0) radius 2.1
  circle A10 centre (97.0443, 0) radius 3 projected
  circle A11 centre (97.0443, 0) radius 2.1
  point P0 (109.0443, -122.0272)
  dimension "d129" = 4.2
  dimension "d130" = 4.2
  dimension "d131" = 4.2
  dimension "d132" = 4.2
  constraints: 4 centre point, 4 coincident
  measures "d129" diameter of A5
  measures "d130" diameter of A7
  measures "d131" diameter of A9
  measures "d132" diameter of A11
extrude "Extrusion22" cut sketch "Sketch22" against normal blind 3 contours A5 | A7 | A9 | A11
sketch "Sketch23" plane through (0, -3, -3) normal (0, 0, -1) x (-1, 0, 0)
  line L0 (-320, 119.0545) -> (-10, 119.0545) construction
  line L1 (0, 69.0244) -> (0, 0) construction
  line L2 (-10, 119.0545) -> (0, 119.0545) construction
  line L3 (0, 119.0545) -> (0, 0) construction
  line L4 (0, 0) -> (-10, 0) construction
  line L5 (-10, 0) -> (-10, 119.0545) construction
  line L6 (-5, 119.0545) -> (-5, 0) construction
  line L7 (0, 0) -> (-320, 0) construction
  circle A0 centre (-5, 104.0545) radius 3
  circle A1 centre (-5, 15) radius 3
  point P0 (0, 3)
  dimension "d135" = 6
  dimension "d136" = 6
  dimension "d137" = 15
  dimension "d138" = 15
  constraints: 10 end point, 3 point on line, 2 centre point, 2 parallel, 2 perpendicular, 1 horizontal, 1 midpoint
  measures "d135" diameter of A0
  measures "d136" diameter of A1
  measures "d137" distance of L6.start A0.centre
  measures "d138" vertical distance of L1.end A1.centre
extrude "Extrusion23" cut sketch "Sketch23" against normal blind 4
sketch "Sketch24" plane through (5, 12, 1) normal (0, 0, -1) x (-1, 0, 0)
  circle A0 centre (0, 0) radius 3 projected
  circle A1 centre (0, 89.0545) radius 3 projected
  circle A2 centre (0, 89.0545) radius 2.1
  circle A3 centre (0, 0) radius 3 projected
  circle A4 centre (0, 0) radius 2.1
  point P0 (5, -12)
  dimension "d141" = 4.2
  dimension "d142" = 4.2
  constraints: 2 centre point, 2 coincident
  measures "d141" diameter of A2
  measures "d142" diameter of A4
extrude "Extrusion24" cut sketch "Sketch24" against normal blind 3 contours A2 | A4
sketch "Sketch25" plane through (330, 0, 0) normal (1, 0, 0) x (0, 0, -1)
  circle A0 centre (-12, 122.0272) radius 3 projected
  circle A1 centre (-109.0443, 122.0272) radius 3 projected
  line L0 (-129.0164, 116.0545) -> (3, 116.0545) projected
  line L1 (3, 116.0545) -> (3, 128) projected
  line L2 (3, 128) -> (-127.4396, 128) projected
  arc A2 (-133.5692, 120.859) -> (-127.4396, 128) centre (-129.0164, 123.1522) ccw projected
  line L3 (-133.5692, 120.859) -> (-135.0362, 119.392) projected
  arc A3 (-135.0362, 119.392) -> (-129.0164, 116.0545) centre (-129.0164, 123.1522) ccw projected
  circle A4 centre (-185.5, 47.9178) radius 3 projected
  circle A5 centre (-185.5, 12) radius 3 projected
  line L4 (-178, -3) -> (-178, 59.8112) projected
  line L5 (-178, 59.8112) -> (-193, 66.0244) projected
  line L6 (-193, 66.0244) -> (-193, -3) projected
  line L7 (-193, -3) -> (-178, -3) projected
  arc A6 (-133.4921, 121.2897) -> (-132.4443, 126.5801) centre (-129.0164, 123.1522) ccw projected
  line L8 (-132.4443, 126.5801) -> (-192.7704, 66.254) projected
  line L9 (-192.7704, 66.254) -> (-189.7704, 65.0114) projected
  line L10 (-189.7704, 65.0114) -> (-133.4921, 121.2897) projected
  point P0 (0, 0)
  point P1 (3, -3)
chamfer "Chamfer1" distance 2 distance2 4 1 edges at (7.5, 5.75, -3) measured on face at (7.5, 6.25, -3)
chamfer "Chamfer2" distance 2 distance2 4 1 edges at (7.5, 0.25, -3) measured on face at (7.5, -0.25, -3)
body "Solid1"
